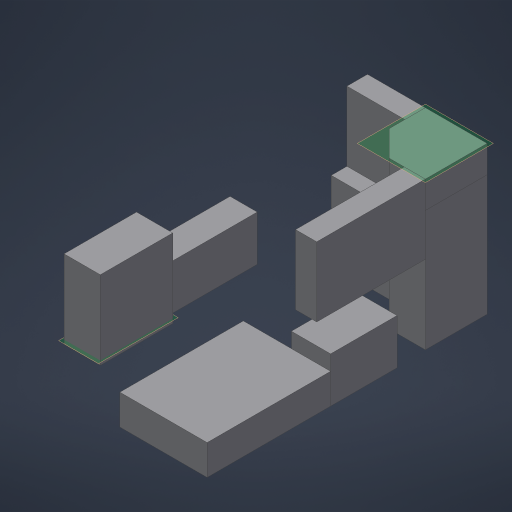
# Autodesk Inventor part: SkeletonLR_00000000
Saved by Autodesk Inventor 2024.3 (Build 283343000, 343)
## iProperties
Created: 2013-04-02
Part Number: SkeletonLR_00000000
Material: Generic
Document SubType Name: Modeling
Designer: User
Density: 1 g/cm^3
Appearance: Default
Description: Darbo Miegamasis kambarys
Author: User
Autodesk Inventor part; units mm, degrees
ref_plane "YZ Plane" through (0, 0, 0) normal (1, 0, 0) x (0, 1, 0)
ref_plane "XZ Plane" through (0, 0, 0) normal (0, 1, 0) x (-1, 0, 0)
ref_plane "XY Plane" through (0, 0, 0) normal (0, 0, 1) x (1, 0, 0)
sketch "Sketch1" plane through (0, 0, 0) normal (0, 0, 1) x (1, 0, 0)
  line L0 (0, 0) -> (3070, 0)
  line L1 (3070, 0) -> (3070, 4940)
  line L2 (3070, 4940) -> (0, 4940)
  line L3 (0, 4940) -> (0, 0)
  line L4 (-250, -250) -> (3320, -250)
  line L5 (3320, -250) -> (3320, 5190)
  line L6 (3320, 5190) -> (-250, 5190)
  line L7 (-250, 5190) -> (-250, -250)
  line L8 (57, 5190) -> (1057, 5190)
  line L9 (1057, 5190) -> (1057, 4940)
  line L10 (1057, 4940) -> (57, 4940)
  line L11 (57, 4940) -> (57, 5190)
  dimension "d0" = 3070
  dimension "d1" = 4940
  dimension "d2" = 250
  dimension "d4" = 2013
  dimension "d5" = 1000
  constraints: 24 end point, 6 parallel, 3 perpendicular, 2 horizontal, 2 point on line, 3 other
  measures "d0" distance of L2.end L1.end
  measures "d1" distance of L1.end L0.end
  measures "d2" distance between parallel lines of L3 L7
  measures "d4" distance between parallel lines of L1 L9
  measures "d5" distance between parallel lines of L9 L11
sketch "Sketch3" plane through (0, 0, 0) normal (0, 0, 1) x (1, 0, 0)
  line L0 (2045.7359, 4340) -> (2470, 3915.7359)
  line L1 (2470, 3915.7359) -> (3070, 3915.7359)
  line L2 (3070, 3915.7359) -> (3070, 4940)
  line L3 (3070, 4940) -> (2045.7359, 4940)
  line L4 (2045.7359, 4940) -> (2045.7359, 4340)
  line L5 (3070, 4940) -> (0, 4940) projected
  line L6 (3070, 0) -> (3070, 4940) projected
  line L7 (2045.7359, 4940) -> (1087, 4940)
  line L8 (1087, 4940) -> (1087, 4340)
  line L9 (1087, 4340) -> (2045.7359, 4340)
  line L10 (2045.7359, 4340) -> (2045.7359, 4940)
  line L11 (1057, 5190) -> (1057, 4940) projected
  point P0 (0, 0)
  dimension "d6" = 45
  dimension "d7" = 600
  dimension "d9" = 600
  dimension "d10" = 30
  constraints: 18 end point, 5 perpendicular, 2 collinear, 2 horizontal, 2 parallel, 1 point on line
  measures "d6" angle of L1 L0
  measures "d7" distance of L0.start L0.end
  measures "d9" distance of L3.end L0.start
  measures "d10" distance between parallel lines of L11 L8
extrude "Extrusion1" add sketch "Sketch3" along normal blind 2000 contours L4 L3 L2 L1 L0
extrude "Extrusion2" add sketch "Sketch3" along normal blind 1300 separate body contours L9 L8 L5 L4
sketch "Sketch4" plane through (0, 0, 2000) normal (0, 0, 1) x (1, 0, 0)
  line L0 (2045.7359, 4340) -> (2470, 3915.7359) projected
  line L1 (2470, 3915.7359) -> (3070, 3915.7359) projected
  line L2 (3070, 3915.7359) -> (3070, 4940) projected
  line L3 (3070, 4940) -> (2045.7359, 4940) projected
  line L4 (2045.7359, 4940) -> (2045.7359, 4340) projected
  point P0 (0, 0)
ref_plane "Work Plane1" through (0, 0, 2450) normal (0, 0, -1) x (-1, 0, 0)
extrude "Extrusion3" add sketch "Sketch4" along normal up to surface (450 mm away) separate body
sketch "Sketch5" plane through (0, 0, 1300) normal (0, 0, 1) x (1, 0, 0)
  line L0 (1087, 4940) -> (1087, 4340) projected
  line L1 (2045.7359, 4940) -> (1087, 4940)
  line L2 (1087, 4940) -> (1087, 4600)
  line L3 (1087, 4600) -> (2045.7359, 4600)
  line L4 (2045.7359, 4600) -> (2045.7359, 4940)
  point P0 (0, 0)
  dimension "d18" = 340
  constraints: 8 end point, 2 parallel, 1 horizontal, 1 perpendicular, 1 point on line
  measures "d18" distance between parallel lines of L1 L3
extrude "Extrusion4" add sketch "Sketch5" along normal up to surface (1150 mm away) bodies 2
sketch "Sketch6" plane through (2470, 3915.7359, 0) normal (0, -1, 0) x (1, 0, 0)
  line L0 (0, 0) -> (600, 0) projected
  line L1 (600, 2450) -> (250, 2450)
  line L2 (250, 2450) -> (250, 1300)
  line L3 (250, 1300) -> (600, 1300)
  line L4 (600, 1300) -> (600, 2450)
  point P0 (-2470, 0)
  dimension "d22" = 1300
  dimension "d23" = 350
  constraints: 8 end point, 2 parallel, 1 horizontal, 1 perpendicular
  measures "d22" distance between parallel lines of L0 L3
  measures "d23" distance of L2.end L3.end
extrude "Extrusion5" add sketch "Sketch6" along normal blind 1800 separate body
sketch "Sketch7" plane through (0, 0, 0) normal (0, 0, 1) x (1, 0, 0)
  line L0 (0, 4940) -> (0, 0) projected
  line L1 (0, 1000) -> (600, 1000)
  line L2 (600, 1000) -> (600, 2200)
  line L3 (600, 2200) -> (0, 2200)
  line L4 (0, 2200) -> (0, 1000)
  line L5 (0, 3750) -> (450, 3750)
  line L6 (450, 3750) -> (450, 2200)
  line L7 (450, 2200) -> (0, 2200)
  line L8 (0, 2200) -> (0, 3750)
  dimension "d26" = 1200
  dimension "d28" = 1550
  dimension "d29" = 450
  dimension "d30" = 600
  dimension "d31" = 1000
  constraints: 16 end point, 4 parallel, 3 point on line, 2 horizontal, 2 perpendicular
  measures "d26" distance between parallel lines of L1 L3
  measures "d28" distance between parallel lines of L5 L3
  measures "d29" distance of L5.start L5.end
  measures "d30" distance of L1.start L1.end
  measures "d31" distance from line of L1 point (0, 0)
extrude "Extrusion6" add sketch "Sketch7" along normal blind 1300 separate body contours L3 L2 L1 L0
extrude "Extrusion7" add sketch "Sketch7" along normal blind 750 separate body contours L5 L6 L3 L0
sketch "Sketch8" plane through (0, 0, 0) normal (0, 0, 1) x (1, 0, 0)
  line L0 (3070, 300) -> (1670, 300) construction
  line L1 (1670, 300) -> (1670, 2300) construction
  line L2 (1670, 2300) -> (3070, 2300) construction
  line L3 (3070, 2300) -> (3070, 300) construction
  line L4 (3070, 3915.7359) -> (3070, 4940) projected
  line L5 (1647, 2323) -> (1647, 277)
  line L6 (1647, 277) -> (3093, 277)
  line L7 (3093, 277) -> (3093, 2323)
  line L8 (3093, 2323) -> (1647, 2323)
  point P0 (0, 0)
  dimension "d36" = 1400
  dimension "d38" = 300
  dimension "d39" = 2000
  dimension "d40" = 23
  constraints: 16 end point, 4 parallel, 2 perpendicular, 1 collinear, 1 horizontal, 3 other
  measures "d36" distance of L1.end L2.end
  measures "d38" distance from line of L0 point (0, 0)
  measures "d39" distance of L0.end L1.end
  measures "d40" distance between parallel lines of L1 L5
extrude "Extrusion8" add sketch "Sketch8" along normal blind 500 separate body
ref_plane "Plintuso aukstis" through (0, 0, 70) normal (0, 0, -1) x (-1, 0, 0)
sketch "Sketch9" plane through (0, 0, 0) normal (0, 0, -1) x (-1, 0, 0)
  line L0 (-3093, 2323) -> (-2443, 2323)
  line L1 (-2443, 2323) -> (-2443, 3423)
  line L2 (-2443, 3423) -> (-3093, 3423)
  line L3 (-3093, 3423) -> (-3093, 2323)
  line L4 (-2470, 3915.7359) -> (-3070, 3915.7359) projected
  point P0 (0, 0)
  dimension "d45" = 1100
  dimension "d47" = 650
  constraints: 8 end point, 2 parallel, 1 horizontal, 1 perpendicular
  measures "d45" distance of L0.end L1.end
  measures "d47" distance of L1.end L2.end
extrude "Extrusion9" add sketch "Sketch9" against normal blind 750 separate body
